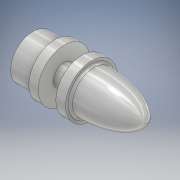
# Autodesk Inventor part: mocowanie_smigla
Saved by Autodesk Inventor 2017 (Build 210142000, 142)
## iProperties
Created: 2017-05-09
Part Number: mocowanie_smigla
Material: Ogólny
Document SubType Name: Modeling
Designer: Kuba01
Density: 1 g/cm^3
Appearance: Domyślna
Author: Kuba01
Autodesk Inventor part; units mm, degrees
ref_plane "YZ Plane" through (0, 0, 0) normal (1, 0, 0) x (0, 1, 0)
ref_plane "XZ Plane" through (0, 0, 0) normal (0, 1, 0) x (-1, 0, 0)
ref_plane "XY Plane" through (0, 0, 0) normal (0, 0, 1) x (1, 0, 0)
sketch "Szkic1" plane through (0, 0, 0) normal (0, 0, 1) x (1, 0, 0)
  line L0 (-24.8894, -0.3525) -> (25.4856, -0.3525)
  line L1 (-22.6958, -0.3525) -> (-22.6958, 4.6475)
  line L2 (-22.6958, 4.6475) -> (-17.6958, 4.6475)
  line L3 (-17.6958, 4.6475) -> (-17.6958, 5.5475)
  line L4 (-17.6958, 5.5475) -> (-15.5558, 5.5475)
  line L5 (-15.5558, 5.5475) -> (-15.5558, 2.0975)
  line L6 (-15.5558, 2.0975) -> (-11.5558, 2.0975)
  line L7 (-11.5558, 2.0975) -> (-11.5558, 5.5475)
  line L8 (-11.5558, 5.5475) -> (-9.3558, 5.5475)
  line L9 (-9.3558, 5.5475) -> (-9.3558, 4.4625)
  line L10 (-9.3558, 4.4625) -> (-3.2506, 4.4625) construction
  line L11 (-3.2506, 4.4625) -> (0.6286, 3.2981) construction
  line L12 (0.6286, 3.2981) -> (3.3042, 1.1615) construction
  line L13 (3.3042, 1.1615) -> (3.3042, -0.3525) construction
  spline S0 degree 4 poles (-9.3558, 4.4625) (-3.2506, 4.4625) (0.6286, 3.2981) (3.3042, 1.1615) (3.3042, -0.3525) knots 1 1 1 1 1 2 2 2 2 2
  point P0 (0, 0)
  point P1 (-16.6258, 5.5475)
  point P2 (-10.4558, 5.5475)
  dimension "d0" = 10
  dimension "d1" = 5
  dimension "d2" = 11.8
  dimension "d3" = 7.14
  dimension "d4" = 4.9
  dimension "d5" = 4
  dimension "d6" = 2.2
  dimension "d7" = 9.63
  dimension "d8" = 26
  constraints: 20 end point, 7 perpendicular, 4 point on line, 2 midpoint, 1 horizontal, 1 horizontal alignment, 1 parallel, 1 vertical, 3 other
  measures "d0" diameter of L2 L0
  measures "d1" distance between parallel lines of L3 L1
  measures "d2" diameter of L4 L0
  measures "d3" distance between parallel lines of L5 L1
  measures "d4" diameter of L6 L0
  measures "d5" distance between parallel lines of L7 L5
  measures "d6" distance between parallel lines of L9 L7
  measures "d7" diameter of L10 L0
  measures "d8" distance from line of L13.end L1
revolve "Obrót1" add sketch "Szkic1" angle 360 about axis through (-24.8894, -0.3525, 0) along (1, 0, 0)
fillet "Zaokrąglenie1" radius 0.5 2 edges at (-9.3558, -5.1675, 0) (-17.6958, -5.3525, 0)
sketch "Szkic2" plane through (-22.6958, -0.3525, 0) normal (-1, 0, 0) x (0, 0, 1)
  point P0 (0, 0.3525)
  point P1 (0, 0.3525)
  constraints: 1 coincident
hole "Otwór1" at (-22.6958, 0, 0) direction (1, 0, 0) diameter 3.11 depth 9 tip angle 118
